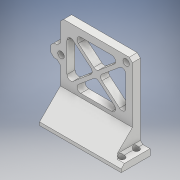
# Autodesk Inventor part: PingCover-y
Saved by Autodesk Inventor 2018.3 (Build 223284000, 284)
## iProperties
Created: 2018-08-25
Part Number: PingCover-y
Material: ABS プラスチック
Document SubType Name: Modeling
Designer: shun2
Density: 1.06 g/cm^3
Appearance: 滑らか - 白
Author: shun2
Autodesk Inventor part; units mm, degrees
ref_plane "YZ Plane" through (0, 0, 0) normal (1, 0, 0) x (0, 1, 0)
ref_plane "XZ Plane" through (0, 0, 0) normal (0, 1, 0) x (-1, 0, 0)
ref_plane "XY Plane" through (0, 0, 0) normal (0, 0, 1) x (1, 0, 0)
sketch "スケッチ1" plane through (0, 0, 0) normal (0, 0, 1) x (1, 0, 0)
  line L0 (0, 0) -> (51, 0)
  line L1 (51, 0) -> (51, 18)
  line L2 (51, 18) -> (0, 18)
  line L3 (0, 18) -> (0, 0)
  circle A0 centre (47, 13.5) radius 1.8
  circle A1 centre (47, 4.5) radius 1.8
  dimension "d0" = 51
  dimension "d1" = 18
  dimension "d4" = 3.6
  dimension "d5" = 13.5
  dimension "d6" = 4
  dimension "d7" = 3.6
  dimension "d8" = 4
  dimension "d9" = 4.5
  constraints: 8 end point, 2 centre point, 2 parallel, 1 horizontal, 1 perpendicular
  measures "d0" distance of L2.end L1.end
  measures "d1" distance of L1.end L0.end
  measures "d4" diameter of A0
  measures "d5" distance from line of L0 A0.centre
  measures "d6" distance from line of L1 A0.centre
  measures "d7" diameter of A1
  measures "d8" distance from line of L1 A1.centre
  measures "d9" distance from line of L0 A1.centre
extrude "押し出し2" add sketch "スケッチ1" along normal blind 2
sketch "スケッチ2" plane through (0, 0, 2) normal (0, 0, 1) x (1, 0, 0)
  line L0 (0, 18) -> (0, 0) projected
  line L1 (0, 18) -> (44, 18)
  line L2 (44, 18) -> (44, 13)
  line L3 (44, 13) -> (0, 13)
  line L4 (0, 13) -> (0, 18)
  dimension "d12" = 44
  dimension "d13" = 5
  constraints: 8 end point, 2 parallel, 1 horizontal, 1 perpendicular
  measures "d12" distance of L2.end L3.end
  measures "d13" distance of L1.end L2.end
extrude "押し出し3" add sketch "スケッチ2" along normal blind 50
sketch "スケッチ3" plane through (0, 13, 2) normal (0, -1, 0) x (1, 0, 0)
  circle A0 centre (41.1, 3.5) radius 2
  line L0 (44, 0) -> (44, 50) projected
  line L1 (44, 0) -> (0, 0) projected
  circle A1 centre (0.4, 19.8) radius 2
  point P0 (0, -2)
  dimension "d16" = 4
  dimension "d17" = 2.9
  dimension "d18" = 3.5
  dimension "d27" = 4
  dimension "d28" = 40.7
  dimension "d29" = 16.3
  constraints: 2 centre point
  measures "d16" diameter of A0
  measures "d17" distance from line of L0 A0.centre
  measures "d18" distance from line of L1 A0.centre
  measures "d27" diameter of A1
  measures "d28" horizontal distance of A0.centre A1.centre
  measures "d29" vertical distance of A0.centre A1.centre
sketch "スケッチ4" plane through (0, 13, 2) normal (0, -1, 0) x (1, 0, 0)
  line L0 (8, 13.3) -> (-4, 13.3)
  line L1 (-4, 13.3) -> (-4, 24.3)
  line L2 (-4, 24.3) -> (8, 24.3)
  line L3 (8, 24.3) -> (8, 13.3)
  line L4 (44, 0) -> (0, 0) projected
  line L5 (44, 0) -> (44, 50) projected
  line L6 (0, 50) -> (44, 50) projected
  line L7 (0, 0) -> (0, 50) projected
  point P0 (0, -2)
  dimension "d19" = 13.3
  dimension "d20" = 36
  dimension "d25" = 11
  dimension "d26" = 12
  constraints: 8 end point, 2 parallel, 1 horizontal, 1 perpendicular
  measures "d19" distance between parallel lines of L0 L4
  measures "d20" distance between parallel lines of L5 L3
  measures "d25" distance between parallel lines of L0 L2
  measures "d26" distance between parallel lines of L1 L3
ref_plane "作業平面2" through (-4, 15.3, 26.3) normal (0, -1, 0) x (1, 0, 0)
sketch "スケッチ5" plane through (-4, 15.3, 26.3) normal (0, -1, 0) x (1, 0, 0)
  point P0 (4, -26.3)
ref_plane "作業平面1" through (-4, 15.3, 26.3) normal (0, -1, 0) x (1, 0, 0)
sketch "スケッチ6" plane through (-4, 15.3, 26.3) normal (0, -1, 0) x (1, 0, 0)
  line L0 (4, -24.3) -> (4, 25.7) projected
  circle A0 centre (4.4, 5.7) radius 2
  circle A1 centre (45.1, 22) radius 2
  line L1 (4, -24.3) -> (55, -24.3) projected
  line L2 (48, -24.3) -> (48, 25.7) projected
  line L3 (4, 25.7) -> (48, 25.7) projected
  point P0 (4, -26.3)
  dimension "d45" = 4
  dimension "d46" = 0.4
  dimension "d47" = 4
  dimension "d48" = 30
  dimension "d49" = 2.9
  dimension "d67" = 43.8427
  constraints: 2 centre point
  measures "d45" diameter of A0
  measures "d46" distance from line of L0 A0.centre
  measures "d47" diameter of A1
  measures "d48" distance from line of L1 A0.centre
  measures "d49" distance from line of L2 A1.centre
  measures "d67" distance of A0.centre A1.centre
sketch "スケッチ7" plane through (0, 13, 2) normal (0, -1, 0) x (1, 0, 0)
  point P0 (0, -2)
sketch "スケッチ8" plane through (0, 13, 2) normal (0, -1, 0) x (1, 0, 0)
  line L0 (44, 0) -> (44, 50) projected
  line L1 (44, 0) -> (45, 0)
  line L2 (45, 0) -> (45, 21.3)
  line L3 (45, 21.3) -> (44, 21.3)
  line L4 (44, 21.3) -> (44, 0)
  point P0 (0, -2)
  dimension "d35" = 1
  constraints: 8 end point, 2 parallel, 1 horizontal, 1 perpendicular
  measures "d35" distance of L3.end L2.end
extrude "押し出し6" add sketch "スケッチ8" against normal blind 5
ref_plane "作業平面3" through (45, 13, 3) normal (0, -1, 0) x (1, 0, 0)
sketch "スケッチ9" plane through (45, 13, 3) normal (0, -1, 0) x (1, 0, 0)
  line L0 (-51, 25.2309) -> (-43, 25.2309)
  line L1 (-43, 25.2309) -> (-43, 33.2309)
  line L2 (-43, 33.2309) -> (-51, 33.2309)
  line L3 (-51, 33.2309) -> (-51, 25.2309)
  line L4 (0, 49) -> (-10, 49)
  line L5 (-10, 49) -> (-10, 15.258)
  line L6 (-10, 15.258) -> (0, 15.258)
  line L7 (0, 15.258) -> (0, 49)
  line L8 (-45, 0) -> (-45, 49) projected
  line L9 (0, 49) -> (-45, 49)
  line L10 (0, 24.7) -> (0, 49)
  point P0 (-45, -3)
  point P1 (-45, 4.4596)
  point P2 (-2.5771, 20.3)
  dimension "d55" = 8
  dimension "d56" = 6
  dimension "d57" = 2
  dimension "d58" = 0
  dimension "d59" = 0
  constraints: 16 end point, 1 horizontal, 1 parallel, 1 vertical, 6 other
  measures "d55" length of L2
  measures "d56" distance between parallel lines of L3 L8
  measures "d57" distance between parallel lines of L8 L1
  measures "d58" vertical extent of L4
  measures "d59" distance between parallel lines of L10 L7
extrude "押し出し8" add sketch "スケッチ9" against normal blind 5
extrude "押し出し9" cut sketch "スケッチ6" along normal mid plane 10 contours A0 L0 | L0 A0 | A1
chamfer "面取り5" distance 13 angle 45 1 edges at (22.5, 13, 2)
sketch "スケッチ10" plane through (0, 0, 2) normal (0, 0, 1) x (1, 0, 0)
  line L0 (45, 18) -> (45, 0) projected
  line L1 (45, 0) -> (51, 0) projected
  line L2 (51, 0) -> (51, 18) projected
  line L3 (51, 18) -> (45, 18) projected
  circle A0 centre (47, 13.5) radius 1.8 projected
  circle A1 centre (47, 4.5) radius 1.8 projected
  circle A2 centre (47, 4.5) radius 1.8
  circle A3 centre (47, 13.5) radius 1.8
  line L4 (45, 0) -> (51, 0)
  line L5 (51, 0) -> (51, 18)
  line L6 (51, 18) -> (45, 18)
  line L7 (45, 18) -> (45, 0)
  point P0 (0, 0)
  constraints: 8 end point, 2 centre point, 2 coincident, 2 concentric, 2 parallel, 1 horizontal, 1 perpendicular
extrude "押し出し10" add sketch "スケッチ10" along normal blind 2
chamfer "面取り6" distance 2 angle 45 1 edges at (48, 0, 4)
chamfer "面取り7" distance 1.5 angle 45 2 edges at (45, 2.0001, 4) (45, 10.0001, 4)
chamfer "面取り8" distance 2 angle 45 4 edges at (45, 15.5, 52) (0, 15.5, 52) (-6, 15.5, 28.2309) (-6, 15.5, 36.2309)
sketch "スケッチ11" plane through (0, 13, 15) normal (0, -1, 0) x (1, 0, 0)
  line L0 (45, 0) -> (45, 35) projected
  line L1 (45, 17.5) -> (40.2419, 17.5)
  line L2 (2, 37) -> (43, 37) projected
  line L3 (19.017, 19.2925) -> (7.9682, 28.5636)
  line L4 (21.1532, 17.5) -> (35.5764, 17.5) construction
  line L5 (19.017, 15.7075) -> (7.9682, 6.4364)
  line L6 (21.1532, 17.5) -> (35.5764, 17.5) construction
  line L7 (4.1241, 8.229) -> (4.1241, 26.771)
  arc A0 (7.9682, 28.5636) -> (4.1241, 26.771) centre (6.4641, 26.771) ccw
  arc A1 (19.017, 15.7075) -> (19.017, 19.2925) centre (17.5129, 17.5) ccw
  arc A2 (4.1241, 8.229) -> (7.9682, 6.4364) centre (6.4641, 8.229) ccw
  line L8 (25.983, 19.2925) -> (37.0318, 28.5636)
  line L9 (25.983, 15.7075) -> (37.0318, 6.4364)
  line L10 (40.8759, 8.229) -> (40.8759, 26.771)
  arc A3 (40.8759, 26.771) -> (37.0318, 28.5636) centre (38.5359, 26.771) ccw
  arc A4 (25.983, 19.2925) -> (25.983, 15.7075) centre (27.4871, 17.5) ccw
  arc A5 (37.0318, 6.4364) -> (40.8759, 8.229) centre (38.5359, 8.229) ccw
  line L11 (23.9337, 20.4379) -> (33.6375, 28.5803)
  line L12 (24.4017, 20.2064) -> (37.0691, 20.2064) construction
  line L13 (20.9255, 20.4379) -> (11.2217, 28.5803)
  line L14 (24.4017, 20.2064) -> (37.0691, 20.2064) construction
  line L15 (12.7258, 32.7129) -> (32.1334, 32.7129)
  arc A6 (20.9255, 20.4379) -> (23.9337, 20.4379) centre (22.4296, 22.2304) ccw
  arc A7 (12.7258, 32.7129) -> (11.2217, 28.5803) centre (12.7258, 30.3729) ccw
  arc A8 (33.6375, 28.5803) -> (32.1334, 32.7129) centre (32.1334, 30.3729) ccw
  line L16 (22.5, 37) -> (22.5, 13.3661)
  line L17 (23.9337, 14.5621) -> (33.6375, 6.4197)
  line L18 (20.9255, 14.5621) -> (11.2217, 6.4197)
  line L19 (12.7258, 2.2871) -> (32.1334, 2.2871)
  arc A9 (23.9337, 14.5621) -> (20.9255, 14.5621) centre (22.4296, 12.7696) ccw
  arc A10 (11.2217, 6.4197) -> (12.7258, 2.2871) centre (12.7258, 4.6271) ccw
  arc A11 (32.1334, 2.2871) -> (33.6375, 6.4197) centre (32.1334, 4.6271) ccw
  point P0 (0, -15)
  point P1 (4.1241, 31.7892)
  point P2 (4.1241, 3.2108)
  point P3 (23.8468, 17.5)
  point P4 (40.8759, 31.7892)
  point P5 (40.8759, 3.2108)
  point P6 (40.5346, 33.7435)
  point P7 (8.2688, 33.7435)
  point P8 (22.5, 17.5)
  dimension "d82" = 22.23
  dimension "d83" = 140
  dimension "d84" = 22.23
  dimension "d85" = 140
  dimension "d86" = 2.34
  dimension "d87" = 21.06
  dimension "d88" = 40
  dimension "d89" = 21.06
  dimension "d90" = 140
  dimension "d91" = 2.34
  constraints: 36 end point, 24 point on circle, 13 point on line, 12 centre point, 12 tangent, 5 horizontal, 4 equal length, 4 equal radius, 2 midpoint, 1 vertical
  measures "d82" distance of L4.start point (4.124, 31.789)
  measures "d83" angle of L4 L3
  measures "d84" distance of L4.start point (4.124, 3.211)
  measures "d85" angle of L5 L6
  measures "d86" radius of A0
  measures "d87" distance of L12.start point (40.535, 33.744)
  measures "d88" angle of L12 L11
  measures "d89" distance of L12.start point (8.269, 33.744)
  measures "d90" angle of L14 L13
  measures "d91" radius of A6
extrude "押し出し11" cut sketch "スケッチ11" against normal blind 5
chamfer "面取り9" distance 2 angle 45 2 edges at (0, 15.5, 36.2309) (0, 15.5, 28.2309)
